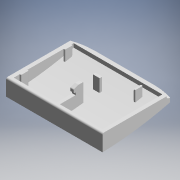
# Autodesk Inventor part: 5395254 CAFC-C6-C
Saved by Autodesk Inventor 2017.3 (Build 213256000, 256)
## iProperties
Part Number: 5395254 CAFC-C6-C
Material: Generic
Catalog Web Link: www.cadenas.de
Description: CAFC-C6-Blind plate
Vendor: FESTO
Document SubType Name: Modeling
Designer: partserver
Manufacturer: FESTO
Mass: 8 g
Surface Area: 58.0874 cm^2
Volume: 5.44266 cm^3
Density: 1 g/cm^3
Appearance: PSOLRGB-255-255-255
Category: PARTsolutions
Company: FESTO
Title: 5395254 CAFC-C6-C
Author: Cadenas PARTsolutions
Comments: Blind plate
PSOL_IDENT_0: {$CADENAS_DATA\23d-libs\festo\parts\c\cafc\cafc_c6.prj},175 {VTYP=3D},{NB=5395254 CAFC-C6-C},{LINA=5
PSOL_IDENT_1: 395254 CAFC-C6-C},{NN=CAFC-C6},{DATE=02.10.2020 11:50:24},{GEOMDATE=14.08.2018 14:25:59},{VERSION=},
PSOL_IDENT_2: {LINEID=10},{WBVAR=},{WBNUMERIC=}  {NB=5395254 CAFC-C6-C},{LINA=5395254 CAFC-C6-C},{KT=DUMMY},{TNR=5
PSOL_IDENT_3: 395254},{TYP=CAFC-C6-C},{CNSMASSEXACT=0.008}
NB: 5395254 CAFC-C6-C
NN: CAFC-C6
NT: Blind plate
NBSYN: $TNR. $TYP.
LINA: 5395254 CAFC-C6-C
CATALOG: Festo
TNR: 5395254
TYP: CAFC-C6-C
CNSMASSEXACT: 0.008
SUPPLIER: FESTO
ARTICLENO: 5395254 CAFC-C6-C
BOMINFO: 5395254 CAFC-C6-C
CREATOR: CADENAS GmbH
Autodesk Inventor part; units mm, degrees
sketch "Sketch_12" plane through (0, 0, 0) normal (1, 0, 0) x (0, 1, 0)
  line L0 (0, 8.5231) -> (0, 0.8)
  arc A0 (0, 0.8) -> (0.8, 0) centre (0.8, 0.8) ccw
  line L1 (0.8, 0) -> (37, 0)
  line L2 (37, 0) -> (37, 2.6942)
  arc A1 (37, 2.6942) -> (36.6281, 3.1775) centre (36.5, 2.6942) ccw
  arc A2 (36.6281, 3.1775) -> (0, 8.5231) centre (-5, -153.9) ccw
  constraints: 6 end point, 6 point on circle, 3 centre point
extrude "Extrusion1" add sketch "Sketch_12" along normal mid plane 50
sketch "Sketch_13" plane through (0, 0, 0) normal (0, 0, 1) x (1, 0, 0)
  line L0 (-28, 32) -> (-25, 32)
  line L1 (-25, 32) -> (-25, 34.807)
  arc A0 (-24.6727, 35.2762) -> (-25, 34.807) centre (-24.5, 34.807) ccw
  arc A1 (-15, 37) -> (-24.6727, 35.2762) centre (-15, 9) ccw
  line L2 (-15, 37) -> (15, 37)
  arc A2 (24.6727, 35.2762) -> (15, 37) centre (15, 9) ccw
  arc A3 (25, 34.807) -> (24.6727, 35.2762) centre (24.5, 34.807) ccw
  line L3 (25, 34.807) -> (25, 32)
  line L4 (25, 32) -> (28, 32)
  line L5 (28, 32) -> (28, 40)
  line L6 (28, 40) -> (-28, 40)
  line L7 (-28, 40) -> (-28, 32)
  constraints: 16 end point, 8 point on circle, 4 centre point
extrude "Extrusion2" cut sketch "Sketch_13" along normal blind 5
sketch "Sketch_2" plane through (0, 0, 0) normal (1, 0, 0) x (0, 1, 0)
  arc A0 (36.671, 1.6084) -> (37, 2.0783) centre (36.5, 2.0783) ccw
  line L0 (36.671, 1.6084) -> (35.658, 1.2397)
  arc A1 (35.658, 1.2397) -> (35, 0.3) centre (36, 0.3) ccw
  line L1 (35, 0.3) -> (35, 0)
  line L2 (35, 0) -> (37, 0)
  line L3 (37, 0) -> (37, 2.0783)
  constraints: 8 end point, 4 point on circle, 2 centre point
extrude "Extrusion3" cut sketch "Sketch_2" along normal mid plane 30
sketch "Sketch_3" plane through (-15, 0, 0) normal (1, 0, 0) x (0, 0, -1)
  line L0 (2.0783, 5.5) -> (0, 5.5)
  arc A0 (-1.6084, 36.671) -> (-2.0783, 37) centre (-2.0783, 36.5) ccw
  line L1 (-1.6084, 36.671) -> (-1.2397, 35.658)
  arc A1 (-1.2397, 35.658) -> (-0.3, 35) centre (-0.3, 36) ccw
  line L2 (-0.3, 35) -> (0, 35)
  line L3 (0, 35) -> (0, 38)
  line L4 (0, 38) -> (-2.0783, 38)
  line L5 (-2.0783, 38) -> (-2.0783, 37)
  constraints: 12 end point, 4 point on circle, 2 centre point
revolve "Revolution1" cut sketch "Sketch_3" angle 30 about axis through (-15, 5.5, -2.0783) along (0, 0, 1)
sketch "Sketch_4" plane through (15, 0, 0) normal (1, 0, 0) x (0, 0, -1)
  line L0 (2.0783, 5.5) -> (0, 5.5)
  arc A0 (-1.6084, 36.671) -> (-2.0783, 37) centre (-2.0783, 36.5) ccw
  line L1 (-1.6084, 36.671) -> (-1.2397, 35.658)
  arc A1 (-1.2397, 35.658) -> (-0.3, 35) centre (-0.3, 36) ccw
  line L2 (-0.3, 35) -> (0, 35)
  line L3 (0, 35) -> (0, 38)
  line L4 (0, 38) -> (-2.0783, 38)
  line L5 (-2.0783, 38) -> (-2.0783, 37)
  constraints: 12 end point, 4 point on circle, 2 centre point
revolve "Revolution2" cut sketch "Sketch_4" angle 30 about axis through (15, 5.5, -2.0783) along (0, 0, -1)
sketch "Sketch_5" plane through (0, 0, 0) normal (1, 0, 0) x (0, 1, 0)
  line L0 (2, 6.4) -> (2, 0)
  line L1 (2, 0) -> (33, 0)
  line L2 (33, 0) -> (33, 2)
  arc A0 (33, 2) -> (2, 6.4) centre (-4.947, -153.9496) ccw
  constraints: 6 end point, 2 point on circle, 1 centre point
extrude "Extrusion4" cut sketch "Sketch_5" along normal mid plane 46
sketch "Sketch_6" plane through (0, 0, 0) normal (1, 0, 0) x (0, 1, 0)
  line L0 (2, 6.55) -> (2, 0)
  line L1 (2, 0) -> (10.125, 0)
  line L2 (10.125, 0) -> (10.125, -1.25)
  line L3 (10.125, -1.25) -> (9.558, -1.25)
  arc A0 (9.558, -1.25) -> (9.3415, -1.375) centre (9.558, -1.5) ccw
  line L4 (9.3415, -1.375) -> (9.1585, -1.692)
  arc A1 (9.1585, -1.692) -> (9.125, -1.817) centre (9.375, -1.817) ccw
  line L5 (9.125, -1.817) -> (9.125, -2.6809)
  arc A2 (9.125, -2.6809) -> (9.454, -3.1507) centre (9.625, -2.6809) ccw
  line L6 (9.454, -3.1507) -> (11.5672, -3.9198)
  arc A3 (11.5672, -3.9198) -> (11.7382, -3.95) centre (11.7382, -3.45) ccw
  line L7 (11.7382, -3.95) -> (13.7, -3.95)
  arc A4 (13.7, -3.95) -> (14.2, -3.45) centre (13.7, -3.45) ccw
  line L8 (14.2, -3.45) -> (14.2, 6.55)
  line L9 (14.2, 6.55) -> (2, 6.55)
  constraints: 20 end point, 10 point on circle, 5 centre point
extrude "Extrusion5" add sketch "Sketch_6" along normal mid plane 1.8
sketch "Sketch_1" plane through (0, 0, -2) normal (0, 0, 1) x (1, 0, 0)
  line L0 (20.3, 6.6) -> (20.3, 3.5)
  arc A0 (20.3, 3.5) -> (20.75, 3.05) centre (20.75, 3.5) ccw
  line L1 (20.75, 3.05) -> (20.85, 3.05)
  arc A1 (20.85, 3.05) -> (21.3, 3.5) centre (20.85, 3.5) ccw
  line L2 (21.3, 3.5) -> (21.3, 6.6)
  arc A2 (21.3, 6.6) -> (20.85, 7.05) centre (20.85, 6.6) ccw
  line L3 (20.85, 7.05) -> (20.75, 7.05)
  arc A3 (20.75, 7.05) -> (20.3, 6.6) centre (20.75, 6.6) ccw
  constraints: 8 end point, 8 point on circle, 4 centre point
extrude "Extrusion6" add sketch "Sketch_1" along normal blind 9
sketch "Sketch_7" plane through (0, 0, -2) normal (0, 0, 1) x (1, 0, 0)
  line L0 (20.3, 29.4) -> (20.3, 26.3)
  arc A0 (20.3, 26.3) -> (20.75, 25.85) centre (20.75, 26.3) ccw
  line L1 (20.75, 25.85) -> (20.85, 25.85)
  arc A1 (20.85, 25.85) -> (21.3, 26.3) centre (20.85, 26.3) ccw
  line L2 (21.3, 26.3) -> (21.3, 29.4)
  arc A2 (21.3, 29.4) -> (20.85, 29.85) centre (20.85, 29.4) ccw
  line L3 (20.85, 29.85) -> (20.75, 29.85)
  arc A3 (20.75, 29.85) -> (20.3, 29.4) centre (20.75, 29.4) ccw
  constraints: 8 end point, 8 point on circle, 4 centre point
extrude "Extrusion7" add sketch "Sketch_7" along normal blind 6
sketch "Sketch_8" plane through (0, 0, -2) normal (0, 0, 1) x (1, 0, 0)
  line L0 (-16.1, 29.4) -> (-16.1, 26.3)
  arc A0 (-16.1, 26.3) -> (-15.65, 25.85) centre (-15.65, 26.3) ccw
  line L1 (-15.65, 25.85) -> (-15.55, 25.85)
  arc A1 (-15.55, 25.85) -> (-15.1, 26.3) centre (-15.55, 26.3) ccw
  line L2 (-15.1, 26.3) -> (-15.1, 29.4)
  arc A2 (-15.1, 29.4) -> (-15.55, 29.85) centre (-15.55, 29.4) ccw
  line L3 (-15.55, 29.85) -> (-15.65, 29.85)
  arc A3 (-15.65, 29.85) -> (-16.1, 29.4) centre (-15.65, 29.4) ccw
  constraints: 8 end point, 8 point on circle, 4 centre point
extrude "Extrusion8" add sketch "Sketch_8" along normal blind 6
sketch "Sketch_9" plane through (0, 0, -2.35) normal (0, 0, 1) x (1, 0, 0)
  line L0 (-1.85, 22.65) -> (-1.85, 22.1)
  arc A0 (-1.85, 22.1) -> (-1.4, 21.65) centre (-1.4, 22.1) ccw
  line L1 (-1.4, 21.65) -> (1.4, 21.65)
  arc A1 (1.4, 21.65) -> (1.85, 22.1) centre (1.4, 22.1) ccw
  line L2 (1.85, 22.1) -> (1.85, 22.65)
  arc A2 (1.85, 22.65) -> (1.4, 23.1) centre (1.4, 22.65) ccw
  line L3 (1.4, 23.1) -> (-1.4, 23.1)
  arc A3 (-1.4, 23.1) -> (-1.85, 22.65) centre (-1.4, 22.65) ccw
  constraints: 8 end point, 8 point on circle, 4 centre point
extrude "Extrusion9" add sketch "Sketch_9" along normal blind 7.35
ref_plane "ANBAU_XY" through (0, 0, 0) normal (0, 1, 0) x (1, 0, 0)
ref_plane "ANBAU_YZ" through (0, 0, 0) normal (1, 0, 0) x (0, 0, -1)
ref_plane "ANBAU_ZX" through (0, 0, 0) normal (0, 0, -1) x (0, 1, 0)
body "Solid1"
